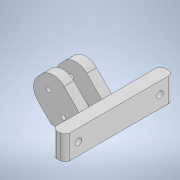
# Autodesk Inventor part: Idle belt holder
Saved by Autodesk Inventor 2022 (Build 260153000, 153)
## iProperties
Created: 2021-10-05
Part Number: Idle belt holder
Material: Generic
Document SubType Name: Modeling
Designer: Administrator
Density: 1 g/cm^3
Appearance: Default
Mass: 4.75917 g
Surface Area: 26.3693 cm^2
Volume: 4.75917 cm^3
Title: Idle belt holder v4
Author: Administrator
Autodesk Inventor part; units mm, degrees
ref_plane "YZ Plane" through (0, 0, 0) normal (1, 0, 0) x (0, 1, 0)
ref_plane "XY Plane" through (0, 0, 0) normal (0, 0, 1) x (1, 0, 0)
ref_plane "Work Plane1" through (0, -6.5, 0) normal (0, 1, 0) x (-1, 0, 0)
sketch "Sketch1" plane through (0, -6.5, 0) normal (0, 1, 0) x (-1, 0, 0)
  line L0 (0, 0) -> (0, 29.475)
  arc A0 (2.625, 32.1) -> (0, 29.475) centre (2.625, 29.475) ccw
  line L1 (7, 29.475) -> (7, 17.5)
  line L2 (22, 12.25) -> (7, 12.25)
  line L3 (2.625, 32.1) -> (4.375, 32.1)
  line L4 (7, 12.25) -> (7, 5.25)
  arc A1 (7, 29.475) -> (4.375, 32.1) centre (4.375, 29.475) ccw
  line L5 (7, 17.5) -> (22, 17.5)
  line L6 (22, 0) -> (0, 0)
  line L7 (7, 5.25) -> (22, 5.25)
  line L8 (0, 0) -> (7, 0)
  line L9 (7, 0) -> (7, -23.825)
  line L10 (4.375, -26.45) -> (2.625, -26.45)
  line L11 (0, -23.825) -> (0, 0)
  arc A2 (0, -23.825) -> (2.625, -26.45) centre (2.625, -23.825) ccw
  arc A3 (4.375, -26.45) -> (7, -23.825) centre (4.375, -23.825) ccw
  line L12 (22, 17.5) -> (22, 12.25)
  line L13 (22, 5.25) -> (22, 0)
  point P0 (0, 0)
  point P1 (7, 0)
  dimension "d35" = 7
  dimension "d36" = 7
  dimension "d38" = 5.25
  dimension "d39" = 14.6
  dimension "d48" = 2.625
  dimension "d49" = 2.625
  dimension "d50" = 23.825
  dimension "d53" = 15
  constraints: 28 end point, 8 point on circle, 8 tangent, 6 horizontal, 5 vertical, 4 centre point, 2 collinear, 2 equal length, 2 equal radius, 2 parallel, 1 coincident, 1 perpendicular
  measures "d35" distance of L2.end L4.end
  measures "d36" distance between parallel lines of L0 L1
  measures "d38" distance between parallel lines of L2 L5
  measures "d39" distance between parallel lines of L3 L5
  measures "d48" radius of A0
  measures "d49" radius of A2
  measures "d50" distance of L8.end L9.end
  measures "d53" distance of L2.start L2.end
extrude "Extrusion2" add sketch "Sketch1" along normal blind 13
hole "Hole3" at (-15.5, 0, 12.25) direction (0, 0, 1) diameter 2.529 depth 5.25 tip angle 118
sketch "Sketch3" plane through (-7, -6.5, 12.25) normal (0, 0, -1) x (-1, 0, 0)
  line L0 (0, 0) -> (0, 13) projected
  line L1 (0, 13) -> (15, 13) projected
  point P0 (8.5, 6.5)
  point P1 (12.375, 13)
  dimension "d51" = 8.5
  dimension "d52" = 6.5
  measures "d51" distance from line of L0 point (8.5, 6.5)
  measures "d52" distance from line of L1 point (8.5, 6.5)
hole "Hole1" at (-15.5, 0, 0) direction (0, 0, 1) diameter 2.529 depth 5.25 tip angle 118
sketch "Sketch6" plane through (-19.375, -6.5, 17.5) normal (0, 0, 1) x (1, 0, 0)
  circle A0 centre (-4.0623, 15.5) radius 4.5
  circle A1 centre (3.875, 6.5) radius 4.5
  circle A2 centre (3.875, 6.5) radius 1.2645 projected
  line L0 (-2.625, 0) -> (12.375, 0) projected
  line L1 (12.375, 0) -> (12.375, 13) projected
  line L2 (-2.625, 13) -> (12.375, 13) projected
  circle A3 centre (3.875, 6.5) radius 1.2645 projected
  circle A4 centre (-4.0623, 15.5) radius 6.5
  circle A5 centre (3.875, 6.5) radius 6.5
  line L3 (3.875, 11) -> (-4.0623, 11)
  line L4 (0, 0) -> (0, 0)
  line L5 (0, 0) -> (0, 13)
  line L6 (0, 13) -> (0, 13)
  line L7 (0, 0) -> (0, 13)
  line L8 (-2.625, 0) -> (-2.625, 13.3311)
  line L9 (-2.625, 0) -> (-15.6685, 13.1351)
  line L10 (-15.6685, 13.1351) -> (-1.6162, 27.0894)
  line L11 (12.375, 0) -> (12.375, 13) projected
  line L12 (-1.6162, 27.0894) -> (12.375, 13)
  line L13 (2.9639, 22.4772) -> (-11.0884, 8.5228)
  circle A6 centre (-4.0623, 15.5) radius 1.2645
  line L14 (-2.625, 0) -> (-2.625, 13) projected
  point P0 (19.375, 6.5)
  point P1 (-2.625, 11)
  point P2 (-0.8154, 11)
  point P3 (-2.625, 1.1851)
  point P4 (3.875, 13)
  point P5 (3.875, 0)
  point P6 (-2.625, 11)
  point P7 (-2.625, 6.5)
  dimension "d26" = 9
  dimension "d27" = 9
  dimension "d28" = 2
  dimension "d29" = 2
  dimension "d30" = 1
  constraints: 12 end point, 3 centre point, 3 horizontal, 2 coincident, 2 perpendicular, 2 point on line, 2 vertical alignment, 1 equal radius, 1 midpoint, 1 parallel, 1 tangent, 1 vertical, 8 other
extrude "Extrusion4" add sketch "Sketch6" against normal up to surface (5.25 mm away) contours A0 L2 L8 L13 A6 | A0 L13 A4 L2 | L13 A6 A0 | A0 L13 A4 | L2 L5 A5 L3 L8 A0 | A0 L8 L2 | A0 L3 L8 A4 L13 | L13 L12 L2 A4 | A4 L10 L12 L13 | L8 L3 A0 | L2 A4 A5 L5 | L13 L9 L10 A4 | A4 L8 L9 L13 | L3 A5 A4 L8 | L2 A5 A4 | L5 L3 A5 | A5 A4 L3 L5 | A4 A5 L8 | L1 L0 A5 L2 | L3 L5 A4 A5 | A5 L5 A1 L3 A4 | L3 A4 L5 | A4 L5 A1 A5 | A5 L5 L0 L8 | L3 A1 L5 A4 | A5 L0 L5 | A1 L5 | L5 A1
ref_plane "Work Plane2" through (-7, -6.5, 8.75) normal (0, 0, -1) x (-1, 0, 0)
mirror "Mirror1" about plane through (-7, -6.5, 8.75) normal (0, 0, -1) of "Extrusion4"
fillet "Fillet1" radius 8.35 4 edges at (-35.0435, 6.6351, 14.875) (-20.9912, 20.5894, 14.875) (-20.9912, 20.5894, 2.625) (-35.0435, 6.6351, 2.625)
sketch "Sketch8" plane through (-7, -6.5, 5.25) normal (-1, 0, 0) x (0, 0, 1)
  line L0 (0, 0) -> (7, 0) projected
  line L1 (7, 0) -> (7, 13) projected
  line L2 (0, 13) -> (7, 13) projected
  line L3 (0, 0) -> (0, 13) projected
  line L4 (12.25, 0) -> (24.225, 0) projected
  line L5 (24.225, 0) -> (24.225, 13) projected
  line L6 (12.25, 13) -> (24.225, 13) projected
  line L7 (12.25, 0) -> (12.25, 13) projected
  line L8 (24.225, 0) -> (26.85, 0) projected
  line L9 (26.85, 0) -> (26.85, 13) projected
  line L10 (24.225, 13) -> (26.85, 13) projected
  line L11 (24.225, 0) -> (24.225, 13) projected
  line L12 (26.85, 0) -> (26.85, 13) construction
  line L13 (26.85, 13) -> (12.25, 0) construction
  point P0 (-5.25, 6.5)
  point P1 (19.55, 6.5)
  point P2 (19.55, 6.5)
  constraints: 2 end point, 1 coincident, 1 midpoint
hole "Hole5" at (-7, 0, 24.8) direction (1, 0, 0) diameter 3.6 end through all counterbore diameter 6.5 counterbore depth 3 clearance for "Socket Head Cap Screw" size "M3" standard "Ansi Metric M Profile"
ref_plane "Work Plane3" through (-2.625, -6.5, 2.825) normal (0, 0, -1) x (-1, 0, 0)
mirror "Mirror2" about plane through (-2.625, -6.5, 2.825) normal (0, 0, -1) of "Hole5"
sketch "Sketch5" plane through (0, -6.5, 0) normal (0, 0, -1) x (-1, 0, 0)
  circle A0 centre (15.5, 6.5) radius 1.2645 projected
  constraints: 1 coincident
ref_plane "Work Plane4" through (-2.625, -6.5, 2.825) normal (0, 0, -1) x (-1, 0, 0)
body "Solid3"
